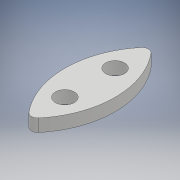
# Autodesk Inventor part: phalanx 3 spring pins support
Saved by Autodesk Inventor 2017 (Build 210142000, 142)
## iProperties
Created: 2018-08-29
Part Number: phalanx 3 spring pins support
Material: Generic
Document SubType Name: Modeling
Designer: jakub.tomczynski
Density: 1 g/cm^3
Appearance: Default
Author: jakub.tomczynski
## iProperties of the stored document phalanx 3 spring pins support_3DPrint.ipt
Created: 2018-09-01
Part Number: phalanx 3 spring pins support_3DPrint
Material: Generic
Document SubType Name: Modeling
Designer: jakub.tomczynski
Density: 1 g/cm^3
Appearance: Default
Author: jakub.tomczynski
Autodesk Inventor part; units mm, degrees
ref_plane "YZ Plane" through (0, 0, 0) normal (1, 0, 0) x (0, 1, 0)
ref_plane "XZ Plane" through (0, 0, 0) normal (0, 1, 0) x (-1, 0, 0)
ref_plane "XY Plane" through (0, 0, 0) normal (0, 0, 1) x (1, 0, 0)
sketch "Sketch2" plane through (0, 0, 0) normal (0, 0, 1) x (1, 0, 0)
  point P0 (0, 0)
  point P1 (-17.5, 0)
  dimension "d6" = 17.5
  constraints: 1 horizontal alignment
  measures "d6" distance of point (0, 0) point (-17.5, 0)
sketch "Sketch1" plane through (0, 0, 0) normal (0, 0, 1) x (1, 0, 0)
  arc A0 (-17.5, -4.899) -> (-17.5, 4.899) centre (-22.5, 0) ccw
  arc A1 (-17.5, 4.899) -> (-17.5, -4.899) centre (-12.5, 0) ccw
  line L0 (-15.5, 0) -> (-15.5, 11.1541) construction
  point P0 (-17.5, 0)
  dimension "d3" = 14
  dimension "d4" = 14
  dimension "d5" = 10
  dimension "d7" = 2
  constraints: 5 point on circle, 2 centre point, 2 end point, 2 horizontal alignment, 1 tangent, 1 vertical
  measures "d3" diameter of A0
  measures "d4" diameter of A1
  measures "d5" distance of A1.centre A0.centre
  measures "d7" distance from line of L0 point (-17.5, 0)
extrude "Extrusion1" add sketch "Sketch1" along normal blind 1
sketch "Sketch3" plane through (0, 0, 1) normal (0, 0, 1) x (1, 0, 0)
  point P0 (0, 0)
  point P1 (-17.5, 0)
  point P2 (-17.5, 2)
  point P3 (-17.5, -2)
  dimension "d10" = 2
  dimension "d11" = 2
  constraints: 2 vertical alignment
  measures "d10" distance of point (-17.5, 2) point (-17.5, 0)
  measures "d11" distance of point (-17.5, 0) point (-17.5, -2)
hole "Hole1" at (-17.5, 2, 1) at (-17.5, -2, 1) direction (0, 0, -1) diameter 1.5 end through all
fillet "Fillet1" radius 0.5 2 edges at (-17.5, -4.899, 0.5) (-17.5, 4.899, 0.5)
body "Solid1"
